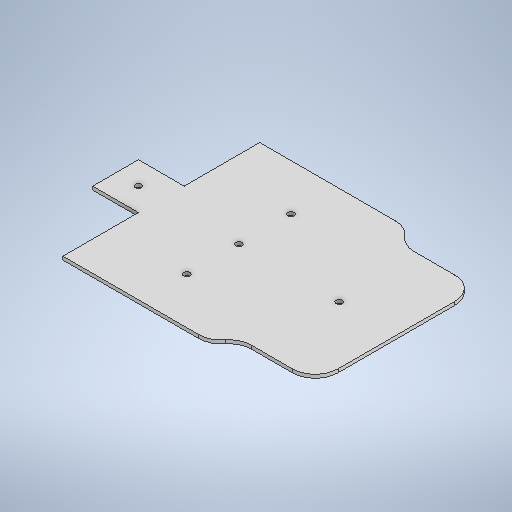
# Autodesk Inventor part: Chassis Front Plate
Saved by Autodesk Inventor 2025.2 (Build 292293000, 293)
## iProperties
Created: 2025-02-20
Part Number: Chassis Front Plate
Material: Generic
Document SubType Name: Modeling
Designer: Matt Tidd
Density: 1 g/cm^3
Appearance: Default
Author: Matt Tidd
Autodesk Inventor part; units mm, degrees
ref_plane "YZ Plane" through (0, 0, 0) normal (1, 0, 0) x (0, 1, 0)
ref_plane "XZ Plane" through (0, 0, 0) normal (0, 1, 0) x (-1, 0, 0)
ref_plane "XY Plane" through (0, 0, 0) normal (0, 0, 1) x (1, 0, 0)
sketch "Sketch1" plane through (0, 0, 0) normal (0, 1, 0) x (-1, 0, 0)
  line L0 (40, 20) -> (80, 20)
  line L1 (80, 20) -> (80, -20)
  line L2 (80, -20) -> (40, -20)
  line L3 (40, -20) -> (40, 20)
  circle A0 centre (60, 0) radius 2.75
  line L4 (40, -86) -> (-165.5, -86)
  line L5 (-165.5, -86) -> (-165.5, 86)
  line L6 (-165.5, 86) -> (40, 86)
  line L7 (40, 86) -> (40, -86)
  line L8 (-165.5, -86) -> (-90.5, -86)
  line L9 (-90.5, -86) -> (-90.5, -71)
  line L10 (-90.5, -71) -> (-165.5, -71)
  line L11 (-165.5, -71) -> (-165.5, -86)
  line L12 (-165.5, 86) -> (-90.5, 86)
  line L13 (-90.5, 86) -> (-90.5, 71)
  line L14 (-90.5, 71) -> (-165.5, 71)
  line L15 (-165.5, 71) -> (-165.5, 86)
  circle A1 centre (-27.75, 0) radius 2.75
  circle A2 centre (-27.75, 45.5) radius 2.75
  circle A3 centre (-27.75, -45.5) radius 2.75
  circle A4 centre (-115.5, 0) radius 2.75
  point P0 (-165.5, 0)
  dimension "d0" = 40
  dimension "d1" = 40
  dimension "d7" = 5.5
  dimension "d24" = 75
  dimension "d25" = 15
  dimension "d26" = 75
  dimension "d27" = 15
  dimension "d29" = 5.5
  dimension "d30" = 5.5
  dimension "d31" = 5.5
  dimension "d32" = 5.5
  constraints: 32 end point, 8 parallel, 5 centre point, 4 horizontal, 4 perpendicular, 1 point on line
  measures "d0" distance of L1.end L2.end
  measures "d1" distance of L0.end L1.end
  measures "d7" diameter of A0
  measures "d24" distance of L10.end L9.end
  measures "d25" distance of L9.end L8.end
  measures "d26" distance of L13.end L14.end
  measures "d27" distance of L12.end L13.end
  measures "d29" diameter of A1
  measures "d30" diameter of A2
  measures "d31" diameter of A3
  measures "d32" diameter of A4
extrude "Extrusion1" add sketch "Sketch1" along normal blind 3 contours L0 L1 L2 L3 | L3 L7 L4 L9 L10 L5 L14 L13 L6
fillet "Fillet6" radius 20 6 edges at (90.5, 1.5, 86) (90.5, 1.5, 71) (165.5, 1.5, 71) (90.5, 1.5, -86) (90.5, 1.5, -71) (165.5, 1.5, -71)
body "Solid1"
